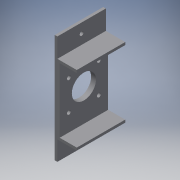
# Autodesk Inventor part: SecondExtruder
Saved by Autodesk Inventor 2016 (Build 200138000, 138)
## iProperties
Created: 2016-05-29
Part Number: SecondExtruder
Material: Generic
Document SubType Name: Modeling
Designer: Scott
Density: 1 g/cm^3
Appearance: Default
Author: Scott
Autodesk Inventor part; units mm, degrees
ref_plane "YZ Plane" through (0, 0, 0) normal (1, 0, 0) x (0, 1, 0)
ref_plane "XZ Plane" through (0, 0, 0) normal (0, 1, 0) x (-1, 0, 0)
ref_plane "XY Plane" through (0, 0, 0) normal (0, 0, 1) x (1, 0, 0)
sketch "Sketch1" plane through (0, 0, 0) normal (0, 0, 1) x (1, 0, 0)
  line L0 (-5.0907, -72.0223) -> (-5.0907, -92.0223) projected
  line L1 (-5.0907, -92.0223) -> (-25.0907, -92.0223) projected
  line L2 (-25.0907, -92.0223) -> (-25.0907, -72.0223) projected
  line L3 (-25.0907, -72.0223) -> (-5.0907, -72.0223) projected
  line L4 (-5.0907, 0) -> (-25.0907, 0) projected
  line L5 (-25.0907, 0) -> (-25.0907, 20) projected
  line L6 (-25.0907, 20) -> (-5.0907, 20) projected
  line L7 (-5.0907, 20) -> (-5.0907, 0) projected
  line L8 (-22.7107, -2.7) -> (-2.3907, -2.7) projected
  line L9 (-2.3907, -2.7) -> (-2.3907, 22.7) projected
  line L10 (-2.3907, 22.7) -> (-27.7907, 22.7) projected
  line L11 (-27.7907, 22.7) -> (-27.7907, -94.7223) projected
  line L12 (-27.7907, -94.7223) -> (-2.3907, -94.7223) projected
  line L13 (-2.3907, -94.7223) -> (-2.3907, -69.3223) projected
  line L14 (-2.3907, -69.3223) -> (-22.7107, -69.3223) projected
  line L15 (-22.7107, -2.7) -> (-22.7107, -69.3223) projected
  line L16 (-25.0907, 20) -> (-25.0907, 22.7)
  line L17 (-22.7107, -2.7) -> (-22.7107, 0)
  line L18 (-22.7107, -69.3223) -> (-22.7107, -72.0223)
  line L19 (-25.0907, -92.0223) -> (-27.7907, -92.0223)
  line L20 (-25.0907, 20) -> (-27.7907, 20)
  line L21 (-5.0907, 0) -> (-5.0907, -2.7)
  line L22 (-5.0907, -72.0223) -> (-5.0907, -69.3223)
  point P0 (0, 0)
  constraints: 14 end point, 8 point on line, 6 perpendicular
extrude "Extrusion1" add sketch "Sketch1" against normal blind 50 contours L3 L18 L14 L22 | L3 L2 L19 L11 L20 L5 L4 L17 L15 L18 | L17 L4 L21 L8
sketch "Sketch2" plane through (-27.7907, -92.0223, 0) normal (-1, 0, 0) x (0, 0, 1)
  line L0 (0, 112.0223) -> (0, 0) projected
  line L1 (0, 112.0223) -> (-50, 112.0223) projected
  line L2 (-50, 0) -> (-50, 112.0223) projected
  line L3 (0, 0) -> (-50, 0) projected
  circle A0 centre (-25, 56.0111) radius 12.5
  line L4 (-25, 56.0111) -> (-40.5, 56.0111)
  line L5 (-40.5, 56.0111) -> (-40.5, 71.5111)
  circle A1 centre (-40.5, 71.5111) radius 2
  circle A2 centre (-40.5, 40.5111) radius 2
  circle A3 centre (-9.5, 71.5111) radius 2
  circle A4 centre (-9.5, 40.5111) radius 2
  point P0 (0, 92.0223)
  dimension "d2" = 25
  dimension "d3" = 15.5
  dimension "d4" = 15.5
  dimension "d5" = 4
  dimension "d8" = 31
  dimension "d11" = 31
  constraints: 5 centre point, 4 end point, 2 horizontal, 1 coincident, 1 perpendicular, 1 vertical, 6 other
  measures "d2" diameter of A0
  measures "d3" distance of L4.start L4.end
  measures "d4" distance of L4.end L5.end
  measures "d5" diameter of A1
  measures "d8" distance of A1.centre A2.centre
  measures "d11" distance of A1.centre A3.centre
extrude "Extrusion2" cut sketch "Sketch2" against normal blind 50 contours A0 | A1 | A2 | A3 | A4
sketch "Sketch3" plane through (-27.7907, -92.0223, 0) normal (-1, 0, 0) x (0, 0, 1)
  circle A0 centre (-9.5, 40.5111) radius 2 projected
  circle A1 centre (-40.5, 40.5111) radius 2 projected
  circle A2 centre (-40.5, 71.5111) radius 2 projected
  circle A3 centre (-9.5, 71.5111) radius 2 projected
  circle A4 centre (-25, 56.0111) radius 12.5 projected
  line L0 (0, 112.0223) -> (0, 0) projected
  line L1 (0, 112.0223) -> (-50, 112.0223) projected
  line L2 (-50, 0) -> (-50, 112.0223) projected
  line L3 (0, 0) -> (-50, 0) projected
  line L4 (-619.5788, 92.0223) -> (142.4212, 92.0223) projected
  line L5 (142.4212, 112.0223) -> (142.4212, 92.0223) projected
  line L6 (142.4212, 112.0223) -> (-619.5788, 112.0223) projected
  line L7 (-619.5788, 92.0223) -> (-619.5788, 112.0223) projected
  circle A5 centre (-25, 102.0223) radius 2
  circle A6 centre (-9.5, 40.5111) radius 2 projected
  circle A7 centre (-40.5, 40.5111) radius 2 projected
  circle A8 centre (-40.5, 71.5111) radius 2 projected
  circle A9 centre (-9.5, 71.5111) radius 2 projected
  circle A10 centre (-25, 56.0111) radius 12.5 projected
  line L8 (0, 112.0223) -> (0, 0) projected
  line L9 (0, 112.0223) -> (-50, 112.0223) projected
  line L10 (-50, 0) -> (-50, 112.0223) projected
  line L11 (0, 0) -> (-50, 0) projected
  line L12 (-619.5855, 0) -> (142.4145, 0) projected
  line L13 (142.4145, 20) -> (142.4145, 0) projected
  line L14 (142.4145, 20) -> (-619.5855, 20) projected
  line L15 (-619.5855, 0) -> (-619.5855, 20) projected
  circle A11 centre (-25, 10) radius 2
  point P0 (0, 92.0223)
  dimension "d16" = 4
  dimension "d17" = 4
  constraints: 2 centre point
  measures "d16" diameter of A5
  measures "d17" diameter of A11
extrude "Extrusion3" cut sketch "Sketch3" against normal blind 50 contours A5 | A11
body "Solid1"
